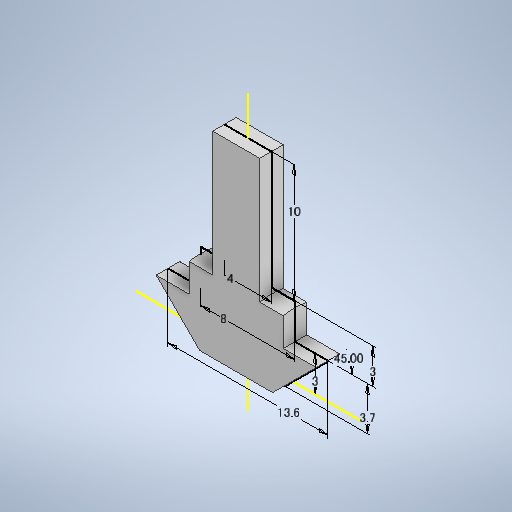
# Autodesk Inventor part: SwitchLeverUnit_Lever
Saved by Autodesk Inventor 2025.1 (Build 291241000, 241)
## iProperties
Created: 2025-03-08
Part Number: SwitchLeverUnit_Lever
Material: 一般
Document SubType Name: Modeling
Designer: kumagai
Density: 1 g/cm^3
Appearance: 既定
Author: kumagai
Autodesk Inventor part; units mm, degrees
ref_plane "YZ Plane" through (0, 0, 0) normal (1, 0, 0) x (0, 1, 0)
ref_plane "XZ Plane" through (0, 0, 0) normal (0, 1, 0) x (-1, 0, 0)
ref_plane "XY Plane" through (0, 0, 0) normal (0, 0, 1) x (1, 0, 0)
sketch "スケッチ1" plane through (0, 0, 0) normal (0, 0, 1) x (1, 0, 0)
  line L0 (0, 19.34) -> (0, -4.04) projected
  line L1 (-9.52, 0) -> (9.52, 0) projected
  line L2 (-6.8, 3) -> (-3.1, -0.7)
  line L3 (-3.1, -0.7) -> (3.1, -0.7)
  line L4 (3.1, -0.7) -> (6.8, 3)
  line L5 (6.8, 3) -> (4, 3)
  line L6 (4, 3) -> (4, 6)
  line L7 (-6.8, 3) -> (-4, 3)
  line L8 (-4, 3) -> (-4, 6)
  line L9 (-4, 6) -> (4, 6)
  line L10 (-2, 6) -> (-2, 16)
  line L11 (-2, 16) -> (2, 16)
  line L12 (2, 16) -> (2, 6)
  point P0 (0, 0)
  dimension "d0" = 13.6
  dimension "d1" = 3
  dimension "d2" = 45
  dimension "d3" = 3.7
  dimension "d4" = 3
  dimension "d5" = 8
  dimension "d6" = 4
  dimension "d7" = 10
  constraints: 22 end point, 6 symmetric about line, 2 horizontal, 2 point on line, 2 vertical
  measures "d0" distance of L4.end L2.start
  measures "d1" distance between parallel lines of L1 L5
  measures "d2" angle of L5 L4
  measures "d3" distance between parallel lines of L3 L5
  measures "d4" distance between parallel lines of L5 L9
  measures "d5" distance between parallel lines of L8 L6
  measures "d6" distance between parallel lines of L10 L12
  measures "d7" distance between parallel lines of L11 L9
extrude "押し出し1" add sketch "スケッチ1" along normal mid plane 2
sketch "スケッチ2" plane through (0, 0, 0) normal (1, 0, 0) x (0, 1, 0)
  line L0 (0, 11.2) -> (0, -11.2) projected
  circle A0 centre (0, 0) radius 5.5
  circle A1 centre (0, 0) radius 8
  point P0 (0, 8)
  point P1 (0, 5.5)
  point P2 (0, -5.5)
  point P3 (0, -8)
  dimension "d10" = 11
  dimension "d11" = 16
  constraints: 2 centre point, 2 coincident
  measures "d10" diameter of A0
  measures "d11" diameter of A1
extrude "押し出し2" cut sketch "スケッチ2" along normal blind 2 from surface at 2 contours A1 L0 A0 picked at (6.7898, -2.1584)
mirror "ミラー1" about plane through (0, 0, 0) normal (1, 0, 0) of "押し出し2"
